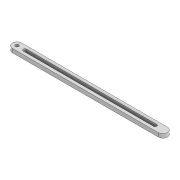
# Autodesk Inventor part: Part_6
Saved by Autodesk Inventor 2022 (Build 260153000, 153)
## iProperties
Created: 2022-04-21
Part Number: Part_6
Material: Generic
Document SubType Name: Modeling
Designer: dell
Density: 1 g/cm^3
Appearance: Default
Author: dell
Autodesk Inventor part; units mm, degrees
ref_plane "YZ Plane" through (0, 0, 0) normal (1, 0, 0) x (0, 1, 0)
ref_plane "XZ Plane" through (0, 0, 0) normal (0, 1, 0) x (-1, 0, 0)
ref_plane "XY Plane" through (0, 0, 0) normal (0, 0, 1) x (1, 0, 0)
sketch "Sketch1" plane through (0, 0, 0) normal (0, 1, 0) x (-1, 0, 0)
  line L0 (0, 0) -> (-188.328, 0) construction
  line L1 (0, 6) -> (-188.328, 6)
  line L2 (-188.328, -6) -> (0, -6)
  arc A0 (0, -6) -> (0, 6) centre (0, 0) ccw
  arc A1 (-188.328, 6) -> (-188.328, -6) centre (-188.328, 0) ccw
  circle A2 centre (0, 0) radius 2.1
  line L3 (-10, 0) -> (-178.328, 0) construction
  line L4 (-10, 2.1) -> (-178.328, 2.1)
  line L5 (-178.328, -2.1) -> (-10, -2.1)
  arc A3 (-10, -2.1) -> (-10, 2.1) centre (-10, 0) ccw
  arc A4 (-178.328, 2.1) -> (-178.328, -2.1) centre (-178.328, 0) ccw
  point P0 (-94.164, 0)
  point P1 (-94.164, 0)
  dimension "d0" = 188.328
  dimension "d1" = 12
  dimension "d2" = 4.2
  dimension "d3" = 4.2
  dimension "d6" = 10
  dimension "d7" = 10
  constraints: 16 end point, 8 point on circle, 8 tangent, 5 centre point, 2 midpoint, 2 parallel, 2 point on line, 1 coincident, 1 horizontal
  measures "d0" distance of L0.end L0.start
  measures "d1" distance between parallel lines of L1 L2
  measures "d2" diameter of A2
  measures "d3" diameter of A4
  measures "d6" distance of L0.start L3.start
  measures "d7" distance of L0.end L3.end
extrude "Extrusion1" add sketch "Sketch1" along normal blind 5
body "Solid1"
